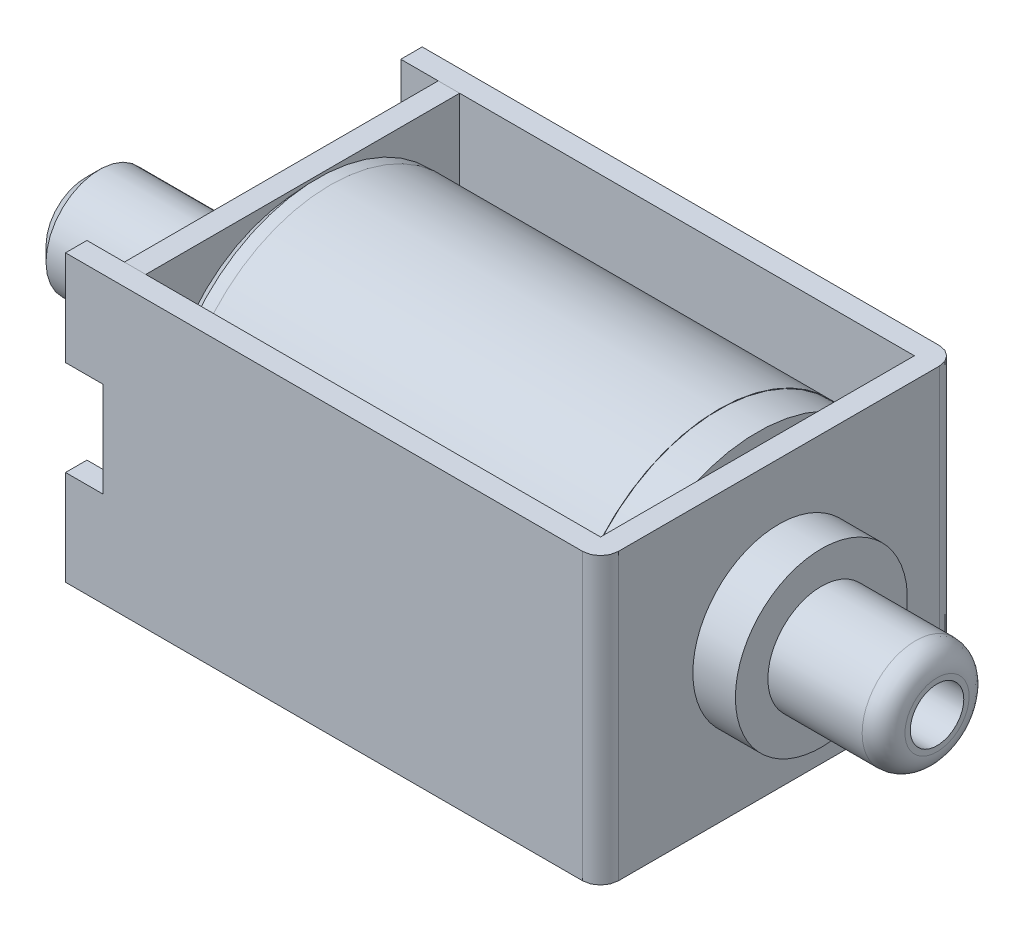
# Autodesk Inventor part: solinoid
Saved by Autodesk Inventor 2022 (Build 260153000, 153)
## iProperties
Created: 2022-06-30
Part Number: solinoid
Material: Generic
Document SubType Name: Modeling
Designer: joshn
Density: 1 g/cm^3
Appearance: Default
Author: joshn
Autodesk Inventor part; units mm, degrees
ref_plane "YZ Plane" through (0, 0, 0) normal (1, 0, 0) x (0, 1, 0)
ref_plane "XZ Plane" through (0, 0, 0) normal (0, 1, 0) x (-1, 0, 0)
ref_plane "XY Plane" through (0, 0, 0) normal (0, 0, 1) x (1, 0, 0)
sketch "Sketch1" plane through (0, 0, 0) normal (0, 1, 0) x (-1, 0, 0)
  line L0 (7.5, 5) -> (-7, 5)
  line L1 (-7.5, 4.5) -> (-7.5, -4.5)
  line L2 (-7, -5) -> (7.5, -5)
  line L3 (7.5, 5) -> (-7.5, -5) construction
  line L4 (-7.5, 5) -> (7.5, -5) construction
  arc A0 (-7, 5) -> (-7.5, 4.5) centre (-7, 4.5) ccw
  arc A1 (-7.5, -4.5) -> (-7, -5) centre (-7, -4.5) ccw
  line L5 (-6.9, 4.4) -> (7.5, 4.4)
  line L6 (7.5, -4.4) -> (-6.9, -4.4)
  line L7 (-6.9, -4.4) -> (-6.9, 4.4)
  line L8 (7.5, -5) -> (7.5, -4.4)
  line L9 (7.5, 4.4) -> (7.5, 5)
  point P0 (0, 0)
  dimension "d0" = 15
  dimension "d1" = 10
  dimension "d2" = 0.5
  dimension "d3" = 0.5
  dimension "d4" = 0.6
  constraints: 20 end point, 4 parallel, 4 point on circle, 4 point on line, 4 tangent, 2 centre point, 2 midpoint, 2 perpendicular, 1 horizontal
  measures "d0" distance of L3.end L2.end
  measures "d1" distance of L4.start L3.end
  measures "d2" radius of A0
  measures "d3" radius of A1
  measures "d4" distance between parallel lines of L0 L5
extrude "Extrusion1" add sketch "Sketch1" along normal blind 8
ref_plane "Work Plane1" through (0, 4, 0) normal (0, 1, 0) x (1, 0, 0)
sketch "Sketch3" plane through (0, 4, 0) normal (0, 1, 0) x (1, 0, 0)
  line L0 (-18.6752, 5.6556) -> (15.176, 5.6556) construction
  line L1 (15.176, 5.6556) -> (15.176, -10.6445) construction
  line L2 (15.176, -10.6445) -> (-18.6752, -10.6445) construction
  line L3 (-18.6752, -10.6445) -> (-18.6752, 5.6556) construction
  point P0 (0, 0)
  point P1 (-7.5, -5)
  constraints: 1 vertical, 3 other
ref_plane "Work Plane2" through (-5.85, 0, -4.4) normal (-1, 0, 0) x (0, 0, 1)
sketch "Sketch4" plane through (-5.85, 0, -4.4) normal (-1, 0, 0) x (0, 0, 1)
  line L0 (8.8, 8) -> (9.4, 8) construction
  line L1 (-0.6, 0) -> (0, 0) construction
  line L2 (0, 0) -> (8.8, 0)
  line L3 (8.8, 0) -> (8.8, 8)
  line L4 (8.8, 8) -> (0, 8)
  line L5 (0, 8) -> (0, 0)
  line L6 (0, 0) -> (0, 8) construction
  line L7 (0, 4) -> (9.4, 4) construction
  line L8 (9.4, 0) -> (9.4, 8) construction
  line L9 (-0.6, 0) -> (-0.6, 8) projected
  line L10 (0.6, 2.6667) -> (-0.6, 2.6667)
  line L11 (-0.6, 2.6667) -> (-0.6, 5.3333)
  line L12 (-0.6, 5.3333) -> (0.6, 5.3333)
  line L13 (0.6, 5.3333) -> (0.6, 2.6667)
  line L14 (0.6, 2.6667) -> (-0.6, 5.3333) construction
  line L15 (-0.6, 2.6667) -> (0.6, 5.3333) construction
  line L16 (4.4, 4) -> (4.4, 7.5833) construction
  line L17 (8.8, 8) -> (8.8, 0)
  line L18 (8.8, 0) -> (8.8, 8) construction
  line L19 (8.8, 4) -> (-0.6, 4) construction
  line L20 (9.4, 0) -> (9.4, 8)
  line L21 (8.2, 2.6667) -> (9.4, 2.6667)
  line L22 (9.4, 2.6667) -> (9.4, 5.3333)
  line L23 (9.4, 5.3333) -> (8.2, 5.3333)
  line L24 (8.2, 5.3333) -> (8.2, 2.6667)
  line L25 (8.2, 2.6667) -> (9.4, 5.3333) construction
  line L26 (9.4, 2.6667) -> (8.2, 5.3333) construction
  point P0 (4.4, 0)
  point P1 (8.8, 2.6667)
  point P2 (8.8, 5.3333)
  point P3 (0, 5.3333)
  point P4 (0, 2.6667)
  dimension "d48" = 2.6667
  dimension "d49" = 8
  constraints: 44 end point, 6 midpoint, 6 symmetric about line, 4 parallel, 3 point on line, 2 horizontal, 2 perpendicular, 1 vertical
  measures "d48" distance of L12.end L10.start
  measures "d49" distance of L1.start L9.end
extrude "Extrusion3" add sketch "Sketch4" along normal blind 0.6 separate body
sketch "Sketch5" plane through (-6.45, 0, -4.4) normal (-1, 0, 0) x (0, 0, 1)
  line L0 (8.8, 0) -> (8.8, 2.6667) projected
  line L1 (8.8, 2.6667) -> (9.4, 2.6667) projected
  line L2 (9.4, 2.6667) -> (9.4, 5.3333) projected
  line L3 (9.4, 5.3333) -> (8.8, 5.3333) projected
  line L4 (8.8, 5.3333) -> (8.8, 8) projected
  line L5 (8.8, 8) -> (0, 8) projected
  line L6 (0, 8) -> (0, 5.3333) projected
  line L7 (0, 5.3333) -> (-0.6, 5.3333) projected
  line L8 (-0.6, 5.3333) -> (-0.6, 2.6667) projected
  line L9 (-0.6, 2.6667) -> (0, 2.6667) projected
  line L10 (0, 2.6667) -> (0, 0) projected
  line L11 (0, 0) -> (8.8, 0) projected
  point P0 (4.4, 0)
extrude "Extrusion4" cut sketch "Sketch5" along normal blind 12.35 bodies 2 1
sketch "Sketch2" plane through (7.5, 0, 4.5) normal (1, 0, 0) x (0, 0, -1)
  line L0 (-0.5, 0) -> (-0.5, 8) construction
  line L1 (-0.5, 4) -> (4.5, 4) construction
  circle A0 centre (4.5, 4) radius 1.5
  point P0 (4.5, 0)
  dimension "d7" = 3
  constraints: 2 end point, 1 centre point, 1 coincident, 1 horizontal, 1 midpoint
  measures "d7" diameter of A0
extrude "Extrusion2" cut sketch "Sketch2" against normal blind 20.75 bodies 1 2
sketch "Sketch7" plane through (0, 4, 0) normal (0, 1, 0) x (1, 0, 0)
  line L0 (1.8647, -1.5) -> (11.9353, -1.5)
  line L1 (11.9353, -1.5) -> (11.9353, 1.5)
  line L2 (11.9353, 1.5) -> (1.8647, 1.5)
  line L3 (1.8647, 1.5) -> (1.8647, -1.5)
  line L4 (6.9, 4.4) -> (6.9, -4.4) projected
  line L5 (1.8647, -1.5) -> (11.9353, 1.5) construction
  line L6 (11.9353, -1.5) -> (1.8647, 1.5) construction
  line L7 (0, 0) -> (11.9353, 0)
  line L8 (1.8647, 0.75) -> (11.9353, 0.75)
  point P0 (6.9, 0)
  point P1 (6.9, 0.75)
  point P2 (6.9, 1.5)
  dimension "d54" = 3
  dimension "d55" = 0.75
  constraints: 16 end point, 4 midpoint, 2 parallel, 2 perpendicular, 2 point on line, 1 horizontal
  measures "d54" distance of L1.end L0.end
  measures "d55" distance between parallel lines of L8 L7
revolve "Revolution1" add sketch "Sketch7" angle 360 about axis through (0, 4, 0) along (1, 0, 0) separate body contours L4 L2 L1 L8
fillet "Fillet1" radius 0.6 1 edges at (11.9353, 4, 1.5)
sketch "Sketch8" plane through (0, 4, 0) normal (0, 1, 0) x (1, 0, 0)
  line L0 (3.0975, 1.5) -> (-11.9475, 1.5)
  line L1 (-11.9475, 1.5) -> (-11.9475, -1.5)
  line L2 (-11.9475, -1.5) -> (3.0975, -1.5)
  line L3 (3.0975, -1.5) -> (3.0975, 1.5)
  line L4 (3.0975, 1.5) -> (-11.9475, -1.5) construction
  line L5 (-11.9475, 1.5) -> (3.0975, -1.5) construction
  line L6 (-0.0808, 0) -> (0, 0)
  line L7 (0, 0) -> (-4.425, 0)
  line L8 (-4.425, 0) -> (-13.7811, 0)
  line L9 (-11.9475, -0.75) -> (3.0975, -0.75)
  dimension "d58" = 3
  dimension "d59" = 0.75
  constraints: 20 end point, 3 point on line, 2 horizontal, 2 midpoint, 2 parallel, 2 perpendicular, 1 collinear
  measures "d58" distance of L1.end L0.end
  measures "d59" distance between parallel lines of L9 L7
revolve "Revolution2" add sketch "Sketch8" angle 360 about axis through (-4.425, 4, 0) along (-1, 0, 0) separate body contours L3 L2 L1 L9
chamfer "Chamfer1" distance 0.4 angle 45 1 edges at (-11.9475, 4, -1.5)
sketch "Sketch9" plane through (0, 4, 0) normal (0, 1, 0) x (1, 0, 0)
  line L0 (0, 0) -> (5.4409, 0)
  line L1 (0, 0) -> (11.9353, 0) projected
  line L2 (-5.0748, -4.3616) -> (5.8144, -4.3616)
  line L3 (5.8144, -4.3616) -> (5.8144, 0)
  line L4 (5.8144, 0) -> (-5.0748, 0)
  line L5 (-5.0748, 0) -> (-5.0748, -4.3616)
  point P0 (2.7204, 0)
  constraints: 10 end point, 2 horizontal, 2 parallel, 1 collinear, 1 perpendicular, 1 point on line
revolve "Revolution3" add sketch "Sketch9" angle 360 about axis through (0, 4, 0) along (1, 0, 0) separate body
sketch "Sketch10" plane through (0, 4, 0) normal (0, 1, 0) x (1, 0, 0)
  line L0 (0, 0) -> (11.9353, 0) projected
  line L1 (0, 0) -> (-15.7999, 0)
  line L2 (6.9, 4.4) -> (6.9, -4.4) projected
  line L3 (5.8144, -4.3477) -> (6.9, -4.3477)
  line L4 (6.9, -4.3477) -> (6.9, 0)
  line L5 (6.9, 0) -> (5.8144, 0)
  line L6 (5.8144, 0) -> (5.8144, -4.3477)
  line L7 (5.8144, 4.3616) -> (5.8144, -4.3616) projected
  line L8 (-5.85, 1.5) -> (-5.85, -1.5) projected
  line L9 (-5.0748, -4.3477) -> (-5.85, -4.3477)
  line L10 (-5.85, -4.3477) -> (-5.85, 0)
  line L11 (-5.85, 0) -> (-5.0748, 0)
  line L12 (-5.0748, 0) -> (-5.0748, -4.3477)
  line L13 (-5.85, -4.4) -> (-5.85, 4.4) projected
  line L14 (-5.85, -3.8909) -> (-5.4281, -4.3477)
  point P0 (6.9, 0)
  point P1 (-5.85, 0)
  constraints: 20 end point, 4 horizontal, 4 parallel, 2 collinear, 2 midpoint, 2 perpendicular, 2 point on line
revolve "Revolution4" add sketch "Sketch10" angle 360 about axis through (0, 4, 0) along (-1, 0, 0) separate body contours L0 L2 L3 L6 | L12 L9 L14 L10 L8 L1
sketch "Sketch11" plane through (0, 4, 0) normal (0, 1, 0) x (1, 0, 0)
  line L0 (7.5, -4.5) -> (7.5, 4.5) projected
  line L1 (7.5, -2.4107) -> (8.6928, -2.4107)
  line L2 (8.6928, -2.4107) -> (8.6928, 0)
  line L3 (8.6928, 0) -> (7.5, 0)
  line L4 (7.5, 0) -> (7.5, -2.4107)
  line L5 (-6.45, -1.5) -> (-6.45, 1.5) projected
  line L6 (-6.45, 0) -> (-7.8782, 0)
  line L7 (-7.8782, 0) -> (-7.8782, -2.4107)
  line L8 (-7.8782, -2.4107) -> (-6.45, -2.4107)
  line L9 (-6.45, -2.4107) -> (-6.45, 0)
  point P0 (0, 0)
  constraints: 16 end point, 4 parallel, 2 horizontal, 2 perpendicular, 2 point on line, 1 midpoint
revolve "Revolution5" add sketch "Sketch11" angle 360 about axis through (-6.45, 4, 0) along (-1, 0, 0) separate body contours L9 L8 L7 L6 L5
revolve "Revolution6" add sketch "Sketch11" angle 360 about axis through (8.6928, 4, 0) along (-1, 0, 0) separate body contours L0 L3 L2 L1
equation "\"d48\" = 0.333333 * d49"
body "Solid1"
body "Solid2"
body "Solid3"
body "Solid4"
body "Solid5"
body "Solid6"
body "Solid7"
body "Solid8"
